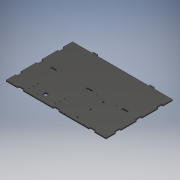
# Autodesk Inventor part: BA02
Saved by Autodesk Inventor 2017 (Build 210142000, 142)
## iProperties
Created: 2019-05-22
Part Number: BA02
Material: Polyethylene, High Density
Document SubType Name: Modeling
Designer: Dell
Density: 0.952 g/cm^3
Appearance: Smooth - Black
Mass: 1092.1 g
Surface Area: 3768.81 cm^2
Volume: 1147.16 cm^3
Author: Dell
Autodesk Inventor part; units mm, degrees
ref_plane "YZ Plane" through (0, 0, 0) normal (1, 0, 0) x (0, 1, 0)
ref_plane "XZ Plane" through (0, 0, 0) normal (0, 1, 0) x (-1, 0, 0)
ref_plane "XY Plane" through (0, 0, 0) normal (0, 0, 1) x (1, 0, 0)
sketch "Sketch1" plane through (0, 0, 0) normal (0, 0, 1) x (1, 0, 0)
  line L0 (0, 0) -> (525.78, 0)
  line L1 (525.78, 0) -> (525.78, 349.25)
  line L2 (525.78, 349.25) -> (0, 349.25)
  line L3 (0, 349.25) -> (0, 0)
  line L4 (239.14, 66.95) -> (239.14, 21.95) construction
  circle A0 centre (239.14, 66.95) radius 2.3813
  circle A1 centre (239.14, 21.95) radius 2.3813
  circle A2 centre (239.14, 44.45) radius 2.3813
  line L5 (179.14, 29.45) -> (179.14, 49.45) construction
  line L6 (169.14, 66.95) -> (169.14, 21.95) construction
  line L7 (179.14, 49.45) -> (159.14, 49.45) construction
  line L8 (159.14, 29.45) -> (179.14, 29.45) construction
  circle A3 centre (169.14, 39.45) radius 10
  line L9 (239.14, 21.95) -> (99.14, 21.95) construction
  line L10 (99.14, 66.95) -> (239.14, 66.95) construction
  line L11 (99.14, 44.45) -> (239.14, 44.45) construction
  line L12 (159.14, 49.45) -> (159.14, 29.45) construction
  line L13 (0, 0) -> (525.78, 0) construction
  line L14 (525.78, 0) -> (525.78, 88.9)
  line L15 (525.78, 88.9) -> (0, 88.9) construction
  line L16 (0, 88.9) -> (0, 0) construction
  line L17 (99.14, 21.95) -> (99.14, 66.95) construction
  circle A4 centre (99.14, 66.95) radius 2.3812
  circle A5 centre (99.14, 21.95) radius 2.3812
  circle A6 centre (99.14, 44.45) radius 2.3812
  point P0 (179.14, 39.45)
  point P1 (159.14, 39.45)
  point P2 (0, 44.45)
  dimension "d0" = 349.25
  dimension "d1" = 525.78
  dimension "d2" = 45
  dimension "d3" = 140
  dimension "d4" = 4.7625
  dimension "d5" = 4.7625
  dimension "d6" = 4.7625
  dimension "d7" = 4.7625
  dimension "d8" = 4.7625
  dimension "d9" = 4.7625
  dimension "d10" = 60
  dimension "d11" = 7.5
  dimension "d12" = 20
  dimension "d13" = 20
  dimension "d15" = 88.9
  dimension "d78" = 169.14
  dimension "d79" = 39.45
  constraints: 36 end point, 8 parallel, 7 midpoint, 6 centre point, 5 coincident, 4 perpendicular, 3 horizontal alignment, 2 horizontal, 2 point on line, 2 other
  measures "d0" distance of L2.end L0.start
  measures "d1" distance of L0.start L0.end
  measures "d2" distance of L4.start L4.end
  measures "d3" distance of L17.end L4.start
  measures "d4" diameter of A4
  measures "d5" diameter of A6
  measures "d6" diameter of A5
  measures "d7" diameter of A1
  measures "d8" diameter of A2
  measures "d9" diameter of A0
  measures "d10" distance from line of L11.end L5
  measures "d11" distance between parallel lines of L9 L8
  measures "d12" distance of L5.end L12.start
  measures "d13" distance of L12.start L8.start
  measures "d15" distance of L15.end L13.start
  measures "d78" distance from line of L3 point (169.14, 39.45)
  measures "d79" distance from line of L0 point (169.14, 39.45)
extrude "Extrusion1" add sketch "Sketch1" along normal blind 6.35
sketch "Sketch2" plane through (0, 0, 6.35) normal (0, 0, 1) x (1, 0, 0)
  line L0 (525.78, 349.25) -> (0, 349.25) projected
  line L1 (101.6, 349.25) -> (127, 349.25)
  line L2 (127, 349.25) -> (127, 355.6)
  line L3 (127, 355.6) -> (101.6, 355.6)
  line L4 (101.6, 355.6) -> (101.6, 349.25)
  line L5 (0, 349.25) -> (0, 0) projected
  line L6 (262.89, 349.25) -> (262.89, 386.8153)
  line L7 (0, 349.25) -> (525.78, 349.25)
  line L8 (424.18, 349.25) -> (398.78, 349.25)
  line L9 (398.78, 349.25) -> (398.78, 355.6)
  line L10 (398.78, 355.6) -> (424.18, 355.6)
  line L11 (424.18, 355.6) -> (424.18, 349.25)
  dimension "d18" = 25.4
  dimension "d19" = 6.35
  dimension "d20" = 101.6
  constraints: 20 end point, 6 symmetric about line, 2 parallel, 2 point on line, 1 horizontal, 1 midpoint, 1 perpendicular, 1 vertical
  measures "d18" distance of L3.end L2.end
  measures "d19" distance of L2.end L1.end
  measures "d20" distance from line of L5 L3.end
extrude "Extrusion2" add sketch "Sketch2" against normal blind 6.35
sketch "Sketch3" plane through (0, 0, 6.35) normal (0, 0, 1) x (1, 0, 0)
  line L0 (101.6, 355.6) -> (101.6, 349.25) projected
  line L1 (127, 355.6) -> (101.6, 355.6) projected
  line L2 (424.18, 355.6) -> (424.18, 349.25) projected
  line L3 (398.78, 355.6) -> (424.18, 355.6) projected
  circle A0 centre (114.3, 352.425) radius 2.25
  circle A1 centre (411.48, 352.425) radius 2.25
  point P0 (0, 0)
  point P1 (114.3, 355.6)
  point P2 (101.6, 352.425)
  point P3 (424.18, 352.425)
  point P4 (411.48, 355.6)
  dimension "d23" = 4.5
  dimension "d24" = 4.5
  constraints: 4 midpoint, 2 centre point, 2 horizontal alignment, 2 vertical alignment
  measures "d23" diameter of A0
  measures "d24" diameter of A1
extrude "Extrusion3" cut sketch "Sketch3" against normal through all
sketch "Sketch4" plane through (0, 0, 6.35) normal (0, 0, 1) x (1, 0, 0)
  line L0 (0, 349.25) -> (0, 0) projected
  line L1 (0, 298.45) -> (6.35, 298.45)
  line L2 (6.35, 298.45) -> (6.35, 273.05)
  line L3 (6.35, 273.05) -> (0, 273.05)
  line L4 (0, 273.05) -> (0, 298.45)
  line L5 (0, 187.325) -> (6.35, 187.325)
  line L6 (6.35, 187.325) -> (6.35, 161.925)
  line L7 (6.35, 161.925) -> (0, 161.925)
  line L8 (0, 161.925) -> (0, 187.325)
  line L9 (0, 50.8) -> (6.35, 50.8)
  line L10 (6.35, 50.8) -> (6.35, 76.2)
  line L11 (6.35, 76.2) -> (0, 76.2)
  line L12 (0, 76.2) -> (0, 50.8)
  line L13 (398.78, 349.25) -> (127, 349.25) projected
  line L14 (262.89, 349.25) -> (262.89, 381.8004)
  line L15 (525.78, 349.25) -> (525.78, 0)
  line L16 (525.78, 298.45) -> (519.43, 298.45)
  line L17 (519.43, 298.45) -> (519.43, 273.05)
  line L18 (519.43, 273.05) -> (525.78, 273.05)
  line L19 (525.78, 273.05) -> (525.78, 298.45)
  line L20 (525.78, 187.325) -> (519.43, 187.325)
  line L21 (519.43, 187.325) -> (519.43, 161.925)
  line L22 (519.43, 161.925) -> (525.78, 161.925)
  line L23 (525.78, 161.925) -> (525.78, 187.325)
  line L24 (525.78, 50.8) -> (519.43, 50.8)
  line L25 (519.43, 50.8) -> (519.43, 76.2)
  line L26 (519.43, 76.2) -> (525.78, 76.2)
  line L27 (525.78, 76.2) -> (525.78, 50.8)
  point P0 (0, 174.625)
  point P1 (525.78, 174.625)
  dimension "d27" = 6.35
  dimension "d28" = 25.4
  dimension "d29" = 6.35
  dimension "d30" = 25.4
  dimension "d31" = 6.35
  dimension "d32" = 25.4
  dimension "d33" = 50.8
  dimension "d34" = 50.8
  constraints: 52 end point, 15 symmetric about line, 6 parallel, 6 point on line, 3 horizontal, 3 midpoint, 3 perpendicular, 1 vertical
  measures "d27" distance of L2.end L3.end
  measures "d28" distance of L1.end L2.end
  measures "d29" distance of L6.end L7.end
  measures "d30" distance of L5.end L6.end
  measures "d31" distance of L11.end L10.end
  measures "d32" distance of L9.end L10.end
  measures "d33" distance from line of L0.start L1
  measures "d34" distance from line of L0.end L9
extrude "Extrusion4" cut sketch "Sketch4" against normal through all
sketch "Sketch5" plane through (0, 0, 0) normal (0, -1, 0) x (1, 0, 0)
  line L0 (62.69, 12.7) -> (88.09, 12.7)
  line L1 (88.09, 12.7) -> (88.09, 0)
  line L2 (88.09, 0) -> (62.69, 0)
  line L3 (62.69, 0) -> (62.69, 12.7)
  line L4 (250.19, 12.7) -> (275.59, 12.7)
  line L5 (275.59, 12.7) -> (275.59, 0)
  line L6 (275.59, 0) -> (250.19, 0)
  line L7 (250.19, 0) -> (250.19, 12.7)
  line L8 (437.69, 12.7) -> (463.09, 12.7)
  line L9 (463.09, 12.7) -> (463.09, 0)
  line L10 (463.09, 0) -> (437.69, 0)
  line L11 (437.69, 0) -> (437.69, 12.7)
  line L12 (75.39, 0) -> (450.39, 0) construction
  line L13 (0, 0) -> (525.78, 0) projected
  point P0 (262.89, 12.7)
  point P1 (262.89, 12.7)
  point P2 (262.89, 0)
  dimension "d37" = 25.4
  dimension "d38" = 12.7
  dimension "d39" = 25.4
  dimension "d40" = 12.7
  dimension "d41" = 25.4
  dimension "d42" = 12.7
  dimension "d43" = 375
  constraints: 26 end point, 6 midpoint, 6 parallel, 3 horizontal, 3 perpendicular, 1 point on line, 1 vertical alignment
  measures "d37" distance of L1.end L2.end
  measures "d38" distance of L1.start L1.end
  measures "d39" distance of L6.start L7.start
  measures "d40" distance of L4.end L6.start
  measures "d41" distance of L9.end L10.end
  measures "d42" distance of L8.end L9.end
  measures "d43" distance of L12.start L12.end
extrude "Extrusion5" cut sketch "Sketch5" against normal blind 6.35
sketch "Sketch6" plane through (0, 0, 6.35) normal (0, 0, 1) x (1, 0, 0)
  line L0 (62.69, 177.325) -> (88.09, 177.325)
  line L1 (88.09, 177.325) -> (88.09, 170.975)
  line L2 (88.09, 170.975) -> (62.69, 170.975)
  line L3 (62.69, 170.975) -> (62.69, 177.325)
  line L4 (250.19, 170.975) -> (275.59, 170.975)
  line L5 (275.59, 170.975) -> (275.59, 177.325)
  line L6 (275.59, 177.325) -> (250.19, 177.325)
  line L7 (250.19, 177.325) -> (250.19, 170.975)
  line L8 (437.69, 170.975) -> (463.09, 170.975)
  line L9 (463.09, 170.975) -> (463.09, 177.325)
  line L10 (463.09, 177.325) -> (437.69, 177.325)
  line L11 (437.69, 177.325) -> (437.69, 170.975)
  line L12 (6.35, 187.325) -> (6.35, 161.925) projected
  line L13 (62.69, 6.35) -> (88.09, 6.35) projected
  line L14 (250.19, 6.35) -> (275.59, 6.35) projected
  line L15 (437.69, 6.35) -> (463.09, 6.35) projected
  point P0 (0, 0)
  dimension "d48" = 6.35
  dimension "d49" = 10
  constraints: 24 end point, 6 parallel, 6 vertical alignment, 3 horizontal, 3 horizontal alignment, 3 perpendicular, 1 point on line
  measures "d48" distance of L0.end L1.end
  measures "d49" distance from line of L12.start L0
extrude "Extrusion6" cut sketch "Sketch6" against normal through all
sketch "Sketch7" plane through (0, 0, 6.35) normal (0, 0, 1) x (1, 0, 0)
  line L0 (275.59, 0) -> (437.69, 0) construction
  line L1 (331.24, 0) -> (382.04, 0) construction
  line L2 (382.04, 0) -> (382.04, 177.325) construction
  line L3 (382.04, 177.325) -> (331.24, 177.325) construction
  line L4 (331.24, 177.325) -> (331.24, 0) construction
  circle A0 centre (356.64, 155.42) radius 4
  circle A1 centre (356.64, 87.71) radius 4
  circle A2 centre (356.64, 20) radius 4
  circle A3 centre (305.84, 174.15) radius 2.25
  circle A4 centre (407.44, 174.15) radius 2.25
  circle A5 centre (305.84, 3.175) radius 2.25
  circle A6 centre (407.44, 3.175) radius 2.25
  line L5 (275.59, 6.35) -> (275.59, 0) projected
  line L6 (437.69, 170.975) -> (437.69, 177.325) projected
  point P0 (0, 0)
  point P1 (275.59, 177.325)
  point P2 (356.64, 0)
  point P3 (356.64, 177.325)
  point P4 (382.04, 88.6625)
  point P5 (275.59, 3.175)
  point P6 (437.69, 174.15)
  dimension "d50" = 50.8
  dimension "d51" = 8
  dimension "d52" = 8
  dimension "d53" = 8
  dimension "d55" = 20
  dimension "d72" = 4.5
  dimension "d73" = 4.5
  dimension "d74" = 4.5
  dimension "d75" = 4.5
  dimension "d76" = 25.4
  dimension "d77" = 25.4
  dimension "d149" = 67.71
  dimension "d150" = 67.71
  constraints: 8 end point, 7 centre point, 6 midpoint, 5 horizontal alignment, 5 vertical alignment, 2 parallel, 1 horizontal, 1 perpendicular, 1 point on line
  measures "d50" distance of L3.end L2.end
  measures "d51" diameter of A0
  measures "d52" diameter of A1
  measures "d53" diameter of A2
  measures "d55" distance from line of L0 A2.centre
  measures "d72" diameter of A3
  measures "d73" diameter of A4
  measures "d74" diameter of A5
  measures "d75" diameter of A6
  measures "d76" distance from line of A3.centre L4
  measures "d77" distance from line of A4.centre L2
  measures "d149" distance of A0.centre A1.centre
  measures "d150" distance of A2.centre A1.centre
extrude "Extrusion7" cut sketch "Sketch7" against normal through all
sketch "Sketch11" plane through (0, 0, 6.35) normal (0, 0, 1) x (1, 0, 0)
  line L0 (0, 50.8) -> (0, 0) projected
  line L1 (0, 49.53) -> (7.62, 49.53)
  line L2 (7.62, 49.53) -> (7.62, 77.47)
  line L3 (7.62, 77.47) -> (0, 77.47)
  line L4 (0, 77.47) -> (0, 49.53)
  line L5 (0, 161.925) -> (0, 76.2) projected
  line L6 (0, 160.655) -> (7.62, 160.655)
  line L7 (7.62, 160.655) -> (7.62, 188.595)
  line L8 (7.62, 188.595) -> (0, 188.595)
  line L9 (0, 188.595) -> (0, 160.655)
  line L10 (0, 273.05) -> (0, 187.325) projected
  line L11 (0, 271.78) -> (7.62, 271.78)
  line L12 (7.62, 271.78) -> (7.62, 299.72)
  line L13 (7.62, 299.72) -> (0, 299.72)
  line L14 (0, 299.72) -> (0, 271.78)
  line L15 (0, 0) -> (525.78, 0) projected
  line L16 (61.42, 0) -> (89.36, 0)
  line L17 (89.36, 0) -> (89.36, 7.62)
  line L18 (89.36, 7.62) -> (61.42, 7.62)
  line L19 (61.42, 7.62) -> (61.42, 0)
  line L20 (0, 0) -> (525.78, 0) projected
  line L21 (248.92, 0) -> (276.86, 0)
  line L22 (276.86, 0) -> (276.86, 7.62)
  line L23 (276.86, 7.62) -> (248.92, 7.62)
  line L24 (248.92, 7.62) -> (248.92, 0)
  line L25 (275.59, 0) -> (437.69, 0) projected
  line L26 (436.42, 0) -> (464.36, 0)
  line L27 (464.36, 0) -> (464.36, 7.62)
  line L28 (464.36, 7.62) -> (436.42, 7.62)
  line L29 (436.42, 7.62) -> (436.42, 0)
  line L30 (248.92, 169.705) -> (276.86, 169.705)
  line L31 (276.86, 169.705) -> (276.86, 178.595)
  line L32 (276.86, 178.595) -> (248.92, 178.595)
  line L33 (248.92, 178.595) -> (248.92, 169.705)
  line L34 (436.42, 169.705) -> (464.36, 169.705)
  line L35 (464.36, 169.705) -> (464.36, 178.595)
  line L36 (464.36, 178.595) -> (436.42, 178.595)
  line L37 (436.42, 178.595) -> (436.42, 169.705)
  line L38 (525.78, 0) -> (525.78, 50.8) projected
  line L39 (525.78, 49.53) -> (518.16, 49.53)
  line L40 (518.16, 49.53) -> (518.16, 77.47)
  line L41 (518.16, 77.47) -> (525.78, 77.47)
  line L42 (525.78, 77.47) -> (525.78, 49.53)
  line L43 (525.78, 160.655) -> (518.16, 160.655)
  line L44 (518.16, 160.655) -> (518.16, 188.595)
  line L45 (518.16, 188.595) -> (525.78, 188.595)
  line L46 (525.78, 188.595) -> (525.78, 160.655)
  line L47 (525.78, 187.325) -> (525.78, 273.05) projected
  line L48 (525.78, 271.78) -> (518.16, 271.78)
  line L49 (518.16, 271.78) -> (518.16, 299.72)
  line L50 (518.16, 299.72) -> (525.78, 299.72)
  line L51 (525.78, 299.72) -> (525.78, 271.78)
  line L52 (519.43, 50.8) -> (519.43, 76.2) projected
  line L53 (519.43, 161.925) -> (519.43, 187.325) projected
  line L54 (519.43, 273.05) -> (519.43, 298.45) projected
  line L55 (250.19, 170.975) -> (250.19, 177.325) projected
  line L56 (437.69, 170.975) -> (437.69, 177.325) projected
  line L57 (6.35, 187.325) -> (6.35, 161.925) projected
  line L58 (6.35, 76.2) -> (6.35, 50.8) projected
  line L59 (6.35, 298.45) -> (6.35, 273.05) projected
  line L60 (62.69, 6.35) -> (88.09, 6.35) projected
  line L61 (250.19, 6.35) -> (275.59, 6.35) projected
  line L62 (437.69, 6.35) -> (463.09, 6.35) projected
  line L63 (437.69, 177.325) -> (463.09, 177.325) projected
  line L64 (519.43, 187.325) -> (525.78, 187.325) projected
  line L65 (519.43, 76.2) -> (525.78, 76.2) projected
  line L66 (525.78, 273.05) -> (519.43, 273.05) projected
  line L67 (250.19, 0) -> (250.19, 6.35) projected
  line L68 (62.69, 0) -> (62.69, 6.35) projected
  line L69 (275.59, 170.975) -> (250.19, 170.975) projected
  line L70 (61.42, 169.705) -> (89.36, 169.705)
  line L71 (89.36, 169.705) -> (89.36, 178.595)
  line L72 (89.36, 178.595) -> (61.42, 178.595)
  line L73 (61.42, 178.595) -> (61.42, 169.705)
  line L74 (88.09, 170.975) -> (62.69, 170.975) projected
  line L75 (62.69, 170.975) -> (62.69, 177.325) projected
  circle A0 centre (129.2451, 351.4951) radius 3.175
  circle A1 centre (99.3549, 351.4951) radius 3.175
  circle A2 centre (396.5349, 351.4951) radius 3.175
  circle A3 centre (426.4251, 351.4951) radius 3.175
  line L76 (101.6, 349.25) -> (99.3549, 351.4951) construction
  line L77 (101.6, 349.25) -> (101.6, 355.6) projected
  point P0 (88.09, 0)
  point P1 (519.43, 63.5)
  point P2 (518.16, 63.5)
  point P3 (519.43, 174.625)
  point P4 (518.16, 174.625)
  point P5 (519.43, 285.75)
  point P6 (518.16, 285.75)
  point P7 (250.19, 174.15)
  point P8 (248.92, 174.15)
  point P9 (437.69, 174.15)
  point P10 (436.42, 174.15)
  point P11 (6.35, 174.625)
  point P12 (7.62, 174.625)
  point P13 (6.35, 63.5)
  point P14 (7.62, 63.5)
  point P15 (6.35, 285.75)
  point P16 (7.62, 285.75)
  point P17 (75.39, 6.35)
  point P18 (75.39, 7.62)
  point P19 (75.39, 6.35)
  point P20 (262.89, 6.35)
  point P21 (262.89, 7.62)
  point P22 (450.39, 6.35)
  point P23 (450.39, 7.62)
  point P24 (262.89, 170.975)
  point P25 (262.89, 169.705)
  point P26 (75.39, 170.975)
  point P27 (75.39, 169.705)
  point P28 (62.69, 174.15)
  point P29 (61.42, 174.15)
  point P30 (398.78, 349.25)
  point P31 (424.18, 349.25)
  point P32 (127, 349.25)
  dimension "d144" = 6.35
  dimension "d145" = 6.35
  dimension "d146" = 6.35
  dimension "d147" = 6.35
  dimension "d84" = 1.27
  dimension "d85" = 1.27
  dimension "d86" = 1.27
  dimension "d87" = 1.27
  dimension "d88" = 1.27
  dimension "d89" = 1.27
  dimension "d90" = 1.27
  dimension "d91" = 1.27
  dimension "d92" = 1.27
  dimension "d93" = 1.27
  dimension "d94" = 1.27
  dimension "d95" = 1.27
  dimension "d148" = 45
  constraints: 98 end point, 29 midpoint, 24 parallel, 17 point on line, 14 horizontal alignment, 12 horizontal, 12 perpendicular, 9 vertical alignment, 4 coincident, 12 other
  measures "d84" distance between parallel lines of L37 L56
  measures "d85" distance between parallel lines of L36 L63
  measures "d86" distance between parallel lines of L44 L53
  measures "d87" distance between parallel lines of L45 L64
  measures "d88" distance between parallel lines of L41 L65
  measures "d89" distance between parallel lines of L66 L48
  measures "d90" distance between parallel lines of L28 L62
  measures "d91" distance between parallel lines of L24 L67
  measures "d92" distance between parallel lines of L19 L68
  measures "d93" distance between parallel lines of L73 L75
  measures "d94" distance between parallel lines of L70 L74
  measures "d95" distance between parallel lines of L58 L2
  measures "d148" angle of L77 L76
extrude "Extrusion10" cut sketch "Sketch11" against normal through all
sketch "Sketch12" plane through (0, 0, 6.35) normal (0, 0, 1) x (1, 0, 0)
  line L0 (101.6, 355.6) -> (101.6, 349.25) projected
  line L1 (101.6, 355.6) -> (127, 355.6)
  line L2 (127, 355.6) -> (127, 356.87)
  line L3 (127, 356.87) -> (101.6, 356.87)
  line L4 (101.6, 356.87) -> (101.6, 355.6)
  line L5 (398.78, 355.6) -> (424.18, 355.6) projected
  line L6 (398.78, 355.6) -> (424.18, 355.6)
  line L7 (424.18, 355.6) -> (424.18, 356.87)
  line L8 (424.18, 356.87) -> (398.78, 356.87)
  line L9 (398.78, 356.87) -> (398.78, 355.6)
  point P0 (0, 0)
  point P1 (101.6, 347.6625)
  dimension "d132" = 1.27
  constraints: 16 end point, 4 parallel, 2 horizontal, 2 perpendicular, 1 coincident, 1 horizontal alignment
  measures "d132" distance of L3.end L0.start
extrude "Extrusion11" add sketch "Sketch12" against normal up to surface (6.35 mm away) from surface at 0
sketch "Sketch14" plane through (0, 0, 6.35) normal (0, 0, 1) x (1, 0, 0)
  line L0 (101.6, 356.87) -> (127, 356.87) projected
  line L1 (101.6, 356.87) -> (102.235, 356.87)
  line L2 (102.235, 356.87) -> (102.235, 350.1587)
  line L3 (102.235, 350.1587) -> (101.6, 350.1587)
  line L4 (101.6, 350.1587) -> (101.6, 356.87)
  line L5 (127, 356.87) -> (126.365, 356.87)
  line L6 (126.365, 356.87) -> (126.365, 350.1587)
  line L7 (126.365, 350.1587) -> (127, 350.1587)
  line L8 (127, 350.1587) -> (127, 356.87)
  line L9 (398.78, 356.87) -> (424.18, 356.87) projected
  line L10 (398.78, 356.87) -> (399.415, 356.87)
  line L11 (399.415, 356.87) -> (399.415, 350.1587)
  line L12 (399.415, 350.1587) -> (398.78, 350.1587)
  line L13 (398.78, 350.1587) -> (398.78, 356.87)
  line L14 (424.18, 356.87) -> (424.18, 353.7401) projected
  line L15 (424.18, 356.87) -> (423.545, 356.87)
  line L16 (423.545, 356.87) -> (423.545, 350.1587)
  line L17 (423.545, 350.1587) -> (424.18, 350.1587)
  line L18 (424.18, 350.1587) -> (424.18, 356.87)
  arc A0 (97.1099, 349.25) -> (101.6, 353.7401) centre (99.3549, 351.4951) ccw projected
  point P0 (0, 0)
  dimension "d151" = 0.635
  dimension "d152" = 0.635
  dimension "d153" = 0.635
  dimension "d154" = 0.635
  constraints: 32 end point, 8 parallel, 4 horizontal, 4 perpendicular, 3 point on line, 1 point on circle
  measures "d151" distance between parallel lines of L13 L11
  measures "d152" distance between parallel lines of L14 L16
  measures "d153" distance between parallel lines of L8 L6
  measures "d154" distance between parallel lines of L4 L2
extrude "Extrusion12" cut sketch "Sketch14" against normal through all contours L0 L2 A0 L4 | A0 L2 L3 L4 | L0 L8 L7 L6 | L9 L11 L12 L13 | L9 L14 L18 L17 L16
equation "\"d16\" = Panel_Thickness"
equation "\"d19\" = Panel_Thickness"
equation "\"d21\" = Panel_Thickness"
equation "\"d27\" = Panel_Thickness"
equation "\"d29\" = Panel_Thickness"
equation "\"d31\" = Panel_Thickness"
equation "\"d40\" = d38"
equation "\"d42\" = d40"
equation "\"d44\" = Panel_Thickness"
equation "\"d48\" = Panel_Thickness"
equation "\"d144\" = Tool_Dia"
equation "\"d145\" = Tool_Dia"
equation "\"d146\" = Tool_Dia"
equation "\"d147\" = Tool_Dia"
equation "\"d84\" = Fit_Tolerance"
equation "\"d85\" = Fit_Tolerance"
equation "\"d86\" = Fit_Tolerance"
equation "\"d87\" = Fit_Tolerance"
equation "\"d88\" = Fit_Tolerance"
equation "\"d89\" = Fit_Tolerance"
equation "\"d90\" = Fit_Tolerance"
equation "\"d91\" = Fit_Tolerance"
equation "\"d92\" = Fit_Tolerance"
equation "\"d93\" = Fit_Tolerance"
equation "\"d94\" = Fit_Tolerance"
equation "\"d95\" = Fit_Tolerance"
equation "\"d132\" = Fit_Tolerance"
equation "\"d151\" = 0.5 * Fit_Tolerance"
equation "\"d152\" = 0.5 * Fit_Tolerance"
equation "\"d153\" = 0.5 * Fit_Tolerance"
equation "\"d154\" = 0.5 * Fit_Tolerance"
equation "\"Fit_Tolerance\" = 1.27"
equation "\"Panel_Thickness\" = 6.35"
equation "\"Tool_Dia\" = 6.35"
body "Solid1"
